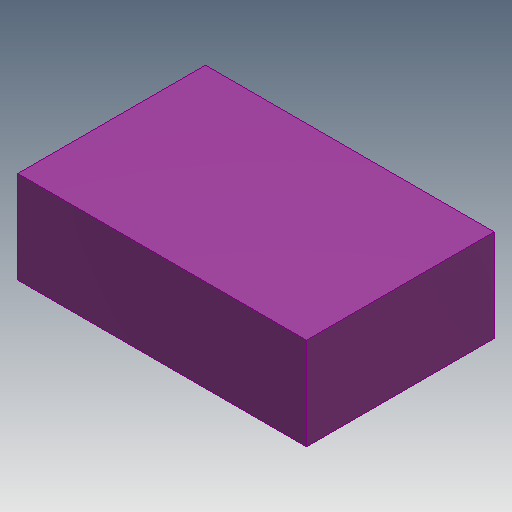
# Autodesk Inventor part: 500MA-PTC
Saved by Autodesk Inventor 2017 (Build 210142000, 142)
## iProperties
Part Number: 500MA-PTC
Material: Generisch
Document SubType Name: Modeling
Designer: Werkstatt
Density: 1 g/cm^3
Appearance: PTC-1206, 500MA-PTC
Author: Werkstatt
Autodesk Inventor part; units mm, degrees
ref_plane "YZ Plane" through (0, 0, 0) normal (1, 0, 0) x (0, 1, 0)
ref_plane "XZ Plane" through (0, 0, 0) normal (0, 1, 0) x (-1, 0, 0)
ref_plane "XY Plane" through (0, 0, 0) normal (0, 0, 1) x (1, 0, 0)
sketch "PTC-1206, 500MA-PTC_13" plane through (0, 0, 0) normal (0, 0, 1) x (1, 0, 0)
  line L0 (-1.5635, 1.016) -> (1.5635, 1.016)
  line L1 (1.5635, 1.016) -> (1.5635, -1.016)
  line L2 (1.5635, -1.016) -> (-1.5635, -1.016)
  line L3 (-1.5635, -1.016) -> (-1.5635, 1.016)
  constraints: 8 end point
extrude "Extrusion1" add sketch "PTC-1206, 500MA-PTC_13" along normal blind 1
